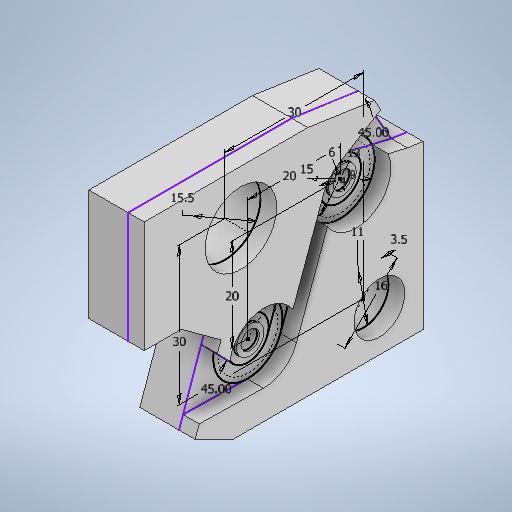
# Autodesk Inventor part: GuideBlock
Saved by Autodesk Inventor 2025.3 (Build 293356030, 356C)
## iProperties
Created: 2025-09-01
Part Number: GuideBlock
Material: Generic
Document SubType Name: Modeling
Designer: tvoko
Density: 1 g/cm^3
Appearance: Default
Author: tvoko
Autodesk Inventor part; units mm, degrees
ref_plane "YZ Plane" through (0, 0, 0) normal (1, 0, 0) x (0, 1, 0)
ref_plane "XZ Plane" through (0, 0, 0) normal (0, 1, 0) x (-1, 0, 0)
ref_plane "XY Plane" through (0, 0, 0) normal (0, 0, 1) x (1, 0, 0)
sketch "Sketch1" plane through (0, 0, 0) normal (1, 0, 0) x (0, 1, 0)
  circle A0 centre (10, -10) radius 2
  circle A1 centre (-10, 10) radius 2
  circle A2 centre (15, 15) radius 7.75
  circle A3 centre (-15, -15) radius 5.5
  line L0 (-9.3431, -20.6569) -> (-20.6569, -9.3431) construction
  circle A4 centre (10, -10) radius 6.5 construction
  circle A5 centre (-10, 10) radius 6.5 construction
  circle A6 centre (-9.3431, -20.6569) radius 1.75
  circle A7 centre (-20.6569, -9.3431) radius 1.75
  line L1 (-10, 10) -> (10, -10) construction
  line L2 (15, 15) -> (-15, -15) construction
  line L3 (11.5041, -24.4668) -> (-23.8171, -24.4668)
  line L4 (-23.8171, -24.4668) -> (-23.8171, 16.7461)
  line L5 (2.4453, 27.8996) -> (26.5977, 27.8996) construction
  line L6 (26.5977, 27.8996) -> (26.5977, 0.4975)
  line L7 (2.4453, 27.8996) -> (-3.8269, 19.3316)
  line L8 (-3.8269, 19.3316) -> (-19.7314, 24.9114)
  line L9 (-19.7314, 24.9114) -> (-23.8171, 16.7461)
  line L10 (11.5041, -24.4668) -> (12, -21.0706)
  line L11 (12, -21.0706) -> (24.4953, -13.9011)
  line L12 (24.4953, -13.9011) -> (26.5977, 0.4975)
  circle A8 centre (10, -10) radius 7.5
  circle A9 centre (-10, 10) radius 7.5
  circle A10 centre (-10, 10) radius 4.5
  circle A11 centre (10, -10) radius 4.5
  line L13 (-11.5314, 5.7686) -> (12.5523, -2.9477)
  line L14 (11.5314, -5.7686) -> (-12.5523, 2.9477)
  line L15 (-13.1242, 13.2387) -> (-6.0131, 20.0985)
  line L16 (-17.4988, 10.1349) -> (-17.2487, 24.0403)
  line L17 (14.3786, -11.0381) -> (12, -21.0706)
  line L18 (16.3837, -6.0632) -> (22.0741, -15.2904)
  circle A12 centre (10, -10) radius 3
  circle A13 centre (-10, 10) radius 3
  line L19 (2.4453, 27.8996) -> (2.4453, 35.9374)
  line L20 (2.4453, 35.9374) -> (26.5977, 35.9374)
  line L21 (26.5977, 35.9374) -> (26.5977, 27.8996)
  point P0 (0, 0)
  point P1 (0, 0)
  point P2 (12.9944, -16.8763)
  point P3 (5.8895, -3.7267)
  point P4 (-8.806, 17.4043)
  point P5 (-5.8895, 3.7267)
  dimension "d0" = 4
  dimension "d2" = 13
  dimension "d3" = 16
  dimension "d4" = 11
  dimension "d5" = 3.5
  dimension "d6" = 20
  dimension "d7" = 20
  dimension "d8" = 30
  dimension "d9" = 30
  dimension "d10" = 15.5
  dimension "d13" = 9
  dimension "d14" = 45
  dimension "d15" = 15
  dimension "d16" = 45
  dimension "d19" = 6
  constraints: 45 end point, 14 centre point, 12 coincident, 8 point on circle, 8 tangent, 6 equal radius, 6 perpendicular, 3 midpoint, 3 point on line, 1 horizontal, 1 parallel, 1 vertical
  measures "d0" diameter of A0
  measures "d2" diameter of A4
  measures "d3" distance of L0.start L0.end
  measures "d4" diameter of A3
  measures "d5" diameter of A6
  measures "d6" horizontal distance of A1.centre A0.centre
  measures "d7" horizontal distance of A1.centre A0.centre
  measures "d8" horizontal distance of A3.centre L2.start
  measures "d9" horizontal distance of L2.start A3.centre
  measures "d10" diameter of A2
  measures "d13" diameter of A11
  measures "d14" angle of L16 L15
  measures "d15" diameter of A8
  measures "d16" angle of L17 L18
  measures "d19" diameter of A12
extrude "Extrusion1" add sketch "Sketch1" against normal blind 8.5 contours L3 L4 L9 L8 L16 A9 L14 A8 L17 L10 | L17 A8 L18 L11 | L18 A8 L13 A9 L15 L8 L7 L19 L20 L21 L6 L12 L11 | L17 A11 L14 A8 | A8 L14 A11 L17 | L14 A9 L13 A8 | A11 | L8 L15 A9 L16 | A9 L15 A10 L13 | L13 A10 L15 A9 | A10 | A12 | A13
extrude "Extrusion2" add sketch "Sketch1" along normal blind 3.5 contours A6 | A7 | L3 L4 L9 L8 L16 A9 L14 A8 L17 L10 | L18 A8 L13 A9 L15 L8 L7 L19 L20 L21 L6 L12 L11
extrude "Extrusion3" add sketch "Sketch1" along normal blind 0.5 contours A12 | A13
body "Solid1"
